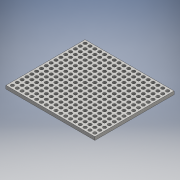
# Autodesk Inventor part: Chassis
Saved by Autodesk Inventor 2016 (Build 200138000, 138)
## iProperties
Created: 2016-05-03
Part Number: Chassis
Material: Generic
Document SubType Name: Modeling
Designer: sunilr
Density: 1 g/cm^3
Appearance: Default
Author: sunilr
Autodesk Inventor part; units mm, degrees
ref_plane "YZ Plane" through (0, 0, 0) normal (1, 0, 0) x (0, 1, 0)
ref_plane "XZ Plane" through (0, 0, 0) normal (0, 1, 0) x (-1, 0, 0)
ref_plane "XY Plane" through (0, 0, 0) normal (0, 0, 1) x (1, 0, 0)
sketch "Sketch1" plane through (0, 0, 0) normal (0, 0, 1) x (1, 0, 0)
  line L0 (0, 0) -> (110, 0)
  line L1 (110, 0) -> (110, 98)
  line L2 (110, 98) -> (0, 98)
  line L3 (0, 98) -> (0, 0)
  circle A0 centre (4, 4) radius 2
  circle A1 centre (10, 4) radius 2
  circle A2 centre (16, 4) radius 2
  circle A3 centre (22, 4) radius 2
  circle A4 centre (28, 4) radius 2
  circle A5 centre (34, 4) radius 2
  circle A6 centre (40, 4) radius 2
  circle A7 centre (46, 4) radius 2
  circle A8 centre (52, 4) radius 2
  circle A9 centre (58, 4) radius 2
  circle A10 centre (64, 4) radius 2
  circle A11 centre (70, 4) radius 2
  circle A12 centre (76, 4) radius 2
  circle A13 centre (82, 4) radius 2
  circle A14 centre (88, 4) radius 2
  circle A15 centre (94, 4) radius 2
  circle A16 centre (100, 4) radius 2
  circle A17 centre (106, 4) radius 2
  circle A18 centre (58, 10) radius 2
  circle A19 centre (64, 10) radius 2
  circle A20 centre (70, 10) radius 2
  circle A21 centre (76, 10) radius 2
  circle A22 centre (82, 10) radius 2
  circle A23 centre (88, 10) radius 2
  circle A24 centre (94, 10) radius 2
  circle A25 centre (100, 10) radius 2
  circle A26 centre (52, 10) radius 2
  circle A27 centre (46, 10) radius 2
  circle A28 centre (40, 10) radius 2
  circle A29 centre (34, 10) radius 2
  circle A30 centre (28, 10) radius 2
  circle A31 centre (22, 10) radius 2
  circle A32 centre (16, 10) radius 2
  circle A33 centre (10, 10) radius 2
  circle A34 centre (106, 10) radius 2
  circle A35 centre (4, 10) radius 2
  circle A36 centre (58, 16) radius 2
  circle A37 centre (64, 16) radius 2
  circle A38 centre (70, 16) radius 2
  circle A39 centre (76, 16) radius 2
  circle A40 centre (82, 16) radius 2
  circle A41 centre (88, 16) radius 2
  circle A42 centre (94, 16) radius 2
  circle A43 centre (100, 16) radius 2
  circle A44 centre (52, 16) radius 2
  circle A45 centre (46, 16) radius 2
  circle A46 centre (40, 16) radius 2
  circle A47 centre (34, 16) radius 2
  circle A48 centre (28, 16) radius 2
  circle A49 centre (22, 16) radius 2
  circle A50 centre (16, 16) radius 2
  circle A51 centre (10, 16) radius 2
  circle A52 centre (106, 16) radius 2
  circle A53 centre (4, 16) radius 2
  circle A54 centre (58, 22) radius 2
  circle A55 centre (64, 22) radius 2
  circle A56 centre (70, 22) radius 2
  circle A57 centre (76, 22) radius 2
  circle A58 centre (82, 22) radius 2
  circle A59 centre (88, 22) radius 2
  circle A60 centre (94, 22) radius 2
  circle A61 centre (100, 22) radius 2
  circle A62 centre (52, 22) radius 2
  circle A63 centre (46, 22) radius 2
  circle A64 centre (40, 22) radius 2
  circle A65 centre (34, 22) radius 2
  circle A66 centre (28, 22) radius 2
  circle A67 centre (22, 22) radius 2
  circle A68 centre (16, 22) radius 2
  circle A69 centre (10, 22) radius 2
  circle A70 centre (106, 22) radius 2
  circle A71 centre (4, 22) radius 2
  circle A72 centre (58, 28) radius 2
  circle A73 centre (64, 28) radius 2
  circle A74 centre (70, 28) radius 2
  circle A75 centre (76, 28) radius 2
  circle A76 centre (82, 28) radius 2
  circle A77 centre (88, 28) radius 2
  circle A78 centre (94, 28) radius 2
  circle A79 centre (100, 28) radius 2
  circle A80 centre (52, 28) radius 2
  circle A81 centre (46, 28) radius 2
  circle A82 centre (40, 28) radius 2
  circle A83 centre (34, 28) radius 2
  circle A84 centre (28, 28) radius 2
  circle A85 centre (22, 28) radius 2
  circle A86 centre (16, 28) radius 2
  circle A87 centre (10, 28) radius 2
  circle A88 centre (106, 28) radius 2
  circle A89 centre (4, 28) radius 2
  circle A90 centre (58, 34) radius 2
  circle A91 centre (64, 34) radius 2
  circle A92 centre (70, 34) radius 2
  circle A93 centre (76, 34) radius 2
  circle A94 centre (82, 34) radius 2
  circle A95 centre (88, 34) radius 2
  circle A96 centre (94, 34) radius 2
  circle A97 centre (100, 34) radius 2
  circle A98 centre (52, 34) radius 2
  circle A99 centre (46, 34) radius 2
  circle A100 centre (40, 34) radius 2
  circle A101 centre (34, 34) radius 2
  circle A102 centre (28, 34) radius 2
  circle A103 centre (22, 34) radius 2
  circle A104 centre (16, 34) radius 2
  circle A105 centre (10, 34) radius 2
  circle A106 centre (106, 34) radius 2
  circle A107 centre (4, 34) radius 2
  circle A108 centre (58, 40) radius 2
  circle A109 centre (64, 40) radius 2
  circle A110 centre (70, 40) radius 2
  circle A111 centre (76, 40) radius 2
  circle A112 centre (82, 40) radius 2
  circle A113 centre (88, 40) radius 2
  circle A114 centre (94, 40) radius 2
  circle A115 centre (100, 40) radius 2
  circle A116 centre (52, 40) radius 2
  circle A117 centre (46, 40) radius 2
  circle A118 centre (40, 40) radius 2
  circle A119 centre (34, 40) radius 2
  circle A120 centre (28, 40) radius 2
  circle A121 centre (22, 40) radius 2
  circle A122 centre (16, 40) radius 2
  circle A123 centre (10, 40) radius 2
  circle A124 centre (106, 40) radius 2
  circle A125 centre (4, 40) radius 2
  circle A126 centre (58, 46) radius 2
  circle A127 centre (64, 46) radius 2
  circle A128 centre (70, 46) radius 2
  circle A129 centre (76, 46) radius 2
  circle A130 centre (82, 46) radius 2
  circle A131 centre (88, 46) radius 2
  circle A132 centre (94, 46) radius 2
  circle A133 centre (100, 46) radius 2
  circle A134 centre (52, 46) radius 2
  circle A135 centre (46, 46) radius 2
  circle A136 centre (40, 46) radius 2
  circle A137 centre (34, 46) radius 2
  circle A138 centre (28, 46) radius 2
  circle A139 centre (22, 46) radius 2
  circle A140 centre (16, 46) radius 2
  circle A141 centre (10, 46) radius 2
  circle A142 centre (106, 46) radius 2
  circle A143 centre (4, 46) radius 2
  circle A144 centre (58, 52) radius 2
  circle A145 centre (64, 52) radius 2
  circle A146 centre (70, 52) radius 2
  circle A147 centre (76, 52) radius 2
  circle A148 centre (82, 52) radius 2
  circle A149 centre (88, 52) radius 2
  circle A150 centre (94, 52) radius 2
  circle A151 centre (100, 52) radius 2
  circle A152 centre (52, 52) radius 2
  circle A153 centre (46, 52) radius 2
  circle A154 centre (40, 52) radius 2
  circle A155 centre (34, 52) radius 2
  circle A156 centre (28, 52) radius 2
  circle A157 centre (22, 52) radius 2
  circle A158 centre (16, 52) radius 2
  circle A159 centre (10, 52) radius 2
  circle A160 centre (106, 52) radius 2
  circle A161 centre (4, 52) radius 2
  circle A162 centre (58, 58) radius 2
  circle A163 centre (64, 58) radius 2
  circle A164 centre (70, 58) radius 2
  circle A165 centre (76, 58) radius 2
  circle A166 centre (82, 58) radius 2
  circle A167 centre (88, 58) radius 2
  circle A168 centre (94, 58) radius 2
  circle A169 centre (100, 58) radius 2
  circle A170 centre (52, 58) radius 2
  circle A171 centre (46, 58) radius 2
  circle A172 centre (40, 58) radius 2
  circle A173 centre (34, 58) radius 2
  circle A174 centre (28, 58) radius 2
  circle A175 centre (22, 58) radius 2
  circle A176 centre (16, 58) radius 2
  circle A177 centre (10, 58) radius 2
  circle A178 centre (106, 58) radius 2
  circle A179 centre (4, 58) radius 2
  circle A180 centre (58, 64) radius 2
  circle A181 centre (64, 64) radius 2
  circle A182 centre (70, 64) radius 2
  circle A183 centre (76, 64) radius 2
  circle A184 centre (82, 64) radius 2
  circle A185 centre (88, 64) radius 2
  circle A186 centre (94, 64) radius 2
  circle A187 centre (100, 64) radius 2
  circle A188 centre (52, 64) radius 2
  circle A189 centre (46, 64) radius 2
  circle A190 centre (40, 64) radius 2
  circle A191 centre (34, 64) radius 2
  circle A192 centre (28, 64) radius 2
  circle A193 centre (22, 64) radius 2
  circle A194 centre (16, 64) radius 2
  circle A195 centre (10, 64) radius 2
  circle A196 centre (106, 64) radius 2
  circle A197 centre (4, 64) radius 2
  circle A198 centre (58, 70) radius 2
  circle A199 centre (64, 70) radius 2
  circle A200 centre (70, 70) radius 2
  circle A201 centre (76, 70) radius 2
  circle A202 centre (82, 70) radius 2
  circle A203 centre (88, 70) radius 2
  circle A204 centre (94, 70) radius 2
  circle A205 centre (100, 70) radius 2
  circle A206 centre (52, 70) radius 2
  circle A207 centre (46, 70) radius 2
  circle A208 centre (40, 70) radius 2
  circle A209 centre (34, 70) radius 2
  circle A210 centre (28, 70) radius 2
  circle A211 centre (22, 70) radius 2
  circle A212 centre (16, 70) radius 2
  circle A213 centre (10, 70) radius 2
  circle A214 centre (106, 70) radius 2
  circle A215 centre (4, 70) radius 2
  circle A216 centre (58, 76) radius 2
  circle A217 centre (64, 76) radius 2
  circle A218 centre (70, 76) radius 2
  circle A219 centre (76, 76) radius 2
  circle A220 centre (82, 76) radius 2
  circle A221 centre (88, 76) radius 2
  circle A222 centre (94, 76) radius 2
  circle A223 centre (100, 76) radius 2
  circle A224 centre (52, 76) radius 2
  circle A225 centre (46, 76) radius 2
  circle A226 centre (40, 76) radius 2
  circle A227 centre (34, 76) radius 2
  circle A228 centre (28, 76) radius 2
  circle A229 centre (22, 76) radius 2
  circle A230 centre (16, 76) radius 2
  circle A231 centre (10, 76) radius 2
  circle A232 centre (106, 76) radius 2
  circle A233 centre (4, 76) radius 2
  circle A234 centre (58, 82) radius 2
  circle A235 centre (64, 82) radius 2
  circle A236 centre (70, 82) radius 2
  circle A237 centre (76, 82) radius 2
  circle A238 centre (82, 82) radius 2
  circle A239 centre (88, 82) radius 2
  circle A240 centre (94, 82) radius 2
  circle A241 centre (100, 82) radius 2
  circle A242 centre (52, 82) radius 2
  circle A243 centre (46, 82) radius 2
  circle A244 centre (40, 82) radius 2
  circle A245 centre (34, 82) radius 2
  circle A246 centre (28, 82) radius 2
  circle A247 centre (22, 82) radius 2
  circle A248 centre (16, 82) radius 2
  circle A249 centre (10, 82) radius 2
  circle A250 centre (106, 82) radius 2
  circle A251 centre (4, 82) radius 2
  circle A252 centre (58, 88) radius 2
  circle A253 centre (64, 88) radius 2
  circle A254 centre (70, 88) radius 2
  circle A255 centre (76, 88) radius 2
  circle A256 centre (82, 88) radius 2
  circle A257 centre (88, 88) radius 2
  circle A258 centre (94, 88) radius 2
  circle A259 centre (100, 88) radius 2
  circle A260 centre (52, 88) radius 2
  circle A261 centre (46, 88) radius 2
  circle A262 centre (40, 88) radius 2
  circle A263 centre (34, 88) radius 2
  circle A264 centre (28, 88) radius 2
  circle A265 centre (22, 88) radius 2
  circle A266 centre (16, 88) radius 2
  circle A267 centre (10, 88) radius 2
  circle A268 centre (106, 88) radius 2
  circle A269 centre (4, 88) radius 2
  circle A270 centre (58, 94) radius 2
  circle A271 centre (64, 94) radius 2
  circle A272 centre (70, 94) radius 2
  circle A273 centre (76, 94) radius 2
  circle A274 centre (82, 94) radius 2
  circle A275 centre (88, 94) radius 2
  circle A276 centre (94, 94) radius 2
  circle A277 centre (100, 94) radius 2
  circle A278 centre (52, 94) radius 2
  circle A279 centre (46, 94) radius 2
  circle A280 centre (40, 94) radius 2
  circle A281 centre (34, 94) radius 2
  circle A282 centre (28, 94) radius 2
  circle A283 centre (22, 94) radius 2
  circle A284 centre (16, 94) radius 2
  circle A285 centre (10, 94) radius 2
  circle A286 centre (106, 94) radius 2
  circle A287 centre (4, 94) radius 2
  dimension "d0" = 110
  dimension "d1" = 98
  dimension "d2" = 4
  dimension "d5" = 6
  dimension "d15" = 6
  constraints: 288 centre point, 8 end point, 2 horizontal, 2 parallel, 1 perpendicular, 1 vertical, 574 other
  measures "d0" distance of L2.end L1.end
  measures "d1" distance of L1.end L0.end
  measures "d2" diameter of A0
  measures "d5" distance of A0.centre A1.centre
  measures "d15" distance of A9.centre A18.centre
extrude "Extrusion1" add sketch "Sketch1" along normal blind 4
body "Solid1"
